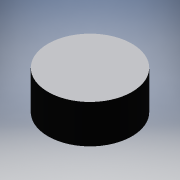
# Autodesk Inventor part: SweepV0.991_BASE_Rev.1
Saved by Autodesk Inventor 2016 (Build 200138000, 138)
## iProperties
Created: 2018-03-01
Part Number: SweepV0.991_BASE_Rev.1
Material: LCP Plastic
Document SubType Name: Modeling
Designer: emvanzant
Density: 1.626 g/cm^3
Appearance: Smooth - White
Author: emvanzant
Autodesk Inventor part; units mm, degrees
ref_plane "YZ Plane" through (0, 0, 0) normal (1, 0, 0) x (0, 1, 0)
sketch "Sketch1" plane through (0, 0, 0) normal (0, 1, 0) x (-1, 0, 0)
  circle A0 centre (0, 0) radius 32.5
  dimension "d0" = 65
  constraints: 1 centre point, 1 coincident
  measures "d0" diameter of A0
extrude "Extrusion1" add sketch "Sketch1" along normal blind 38.5
sketch "Sketch2" plane through (0, 0, 0) normal (0, -1, 0) x (1, 0, 0)
  circle A0 centre (0, 0) radius 25.5
  dimension "d3" = 51
  constraints: 1 centre point, 1 coincident
  measures "d3" diameter of A0
extrude "Extrusion2" add sketch "Sketch2" along normal blind 23.4
chamfer "Chamfer1" distance 3 angle 45 2 edges at (32.5, 38.5, 0) (32.5, 0, 0)
sketch "Sketch3" plane through (0, -23.4, 0) normal (0, -1, 0) x (1, 0, 0)
  line L0 (0, 0) -> (0, -10.5) construction
  circle A0 centre (0, 0) radius 25.5 projected
  line L1 (0, -10.5) -> (5.75, -10.5)
  line L2 (5.75, -10.5) -> (5.75, -24.8433)
  line L3 (0, -10.5) -> (-5.75, -10.5)
  line L4 (-5.75, -10.5) -> (-5.75, -24.8433)
  line L5 (5.75, -24.8433) -> (-5.75, -24.8433)
  line L6 (-15, 15) -> (15, 15) construction
  line L7 (15, 15) -> (15, -15) construction
  line L8 (15, -15) -> (-15, -15) construction
  line L9 (-15, -15) -> (-15, 15) construction
  line L10 (-15, 15) -> (15, -15) construction
  line L11 (15, 15) -> (-15, -15) construction
  line L12 (5.65, 5.65) -> (-5.65, 5.65) construction
  line L13 (-5.65, 5.65) -> (-5.65, -5.65) construction
  line L14 (-5.65, -5.65) -> (5.65, -5.65) construction
  line L15 (5.65, -5.65) -> (5.65, 5.65) construction
  line L16 (5.65, 5.65) -> (-5.65, -5.65) construction
  line L17 (-5.65, 5.65) -> (5.65, -5.65) construction
  dimension "d10" = 10.5
  dimension "d14" = 5.75
  dimension "d15" = 5.75
  dimension "d16" = 30
  dimension "d17" = 30
  dimension "d35" = 11.3
  dimension "d36" = 11.3
  constraints: 36 end point, 8 coincident, 4 horizontal, 4 midpoint, 4 parallel, 4 perpendicular, 2 point on circle, 1 vertical
  measures "d10" distance of L0.start L0.end
  measures "d14" distance of L0.end L1.end
  measures "d15" distance of L0.end L3.end
  measures "d16" distance of L7.end L8.end
  measures "d17" distance of L6.end L7.end
  measures "d35" distance of L14.end L13.end
  measures "d36" distance of L13.end L12.end
hole "Hole1" at (15, -23.4, -15) at (-15, -23.4, -15) at (15, -23.4, 15) at (-15, -23.4, 15) direction (0, 1, 0) diameter 2.5 depth 4
thread "Thread1" size "M2.5x0.45" class "6H" standard "ANSI Metric M Profile" full length
thread "Thread2" size "M2.5x0.45" class "6H" standard "ANSI Metric M Profile" full length
thread "Thread3" size "M2.5x0.45" class "6H" standard "ANSI Metric M Profile" full length
thread "Thread4" size "M2.5x0.45" class "6H" standard "ANSI Metric M Profile" full length
extrude "Extrusion3" cut sketch "Sketch3" against normal blind 12 contours L5 A0 | L4 L3 L1 L2 L5
hole "Hole2" at (5.65, -23.4, 5.65) at (5.65, -23.4, -5.65) at (-5.65, -23.4, 5.65) at (-5.65, -23.4, -5.65) direction (0, 1, 0) diameter 2.1 depth 3 tip angle 118
thread "Thread5" size "M2.5x0.45" class "6H" standard "ANSI Metric M Profile" full length
thread "Thread6" size "M2.2x0.45" class "6H" standard "ANSI Metric M Profile" full length
thread "Thread7" size "M2.2x0.45" class "6H" standard "ANSI Metric M Profile" full length
thread "Thread8" size "M2.2x0.45" class "6H" standard "ANSI Metric M Profile" full length
ref_plane "Work Plane1" through (0, 0, -32.5) normal (0, 0, -1) x (-1, 0, 0)
sketch "Sketch4" plane through (0, 0, -32.5) normal (0, 0, -1) x (-1, 0, 0)
  line L0 (-25.5, -23.4) -> (25.5, -23.4) projected
  line L1 (-32.5, 3) -> (32.5, 3) projected
  line L2 (32.5, 35.5) -> (-32.5, 35.5) projected
  line L3 (0, -23.4) -> (0, 18.1) construction
  line L4 (32.5, 3) -> (32.5, 35.5) projected
  line L5 (-32.5, 3) -> (-32.5, 35.5) projected
  line L6 (-32.5, 17.6) -> (32.5, 17.6)
  line L7 (32.5, 17.6) -> (32.5, 18.6)
  line L8 (32.5, 18.6) -> (-32.5, 18.6)
  line L9 (-32.5, 18.6) -> (-32.5, 17.6)
  line L10 (-32.5, 17.6) -> (32.5, 18.6) construction
  line L11 (32.5, 17.6) -> (-32.5, 18.6) construction
  line L12 (-20, 18.1) -> (20, 18.1) construction
  line L13 (-20, 9.1) -> (20, 9.1)
  line L14 (20, 27.1) -> (-20, 27.1)
  arc A0 (-20, 27.1) -> (-20, 9.1) centre (-20, 18.1) ccw
  arc A1 (20, 9.1) -> (20, 27.1) centre (20, 18.1) ccw
  line L15 (0, 18.1) -> (-15, 18.1)
  line L16 (0, 18.1) -> (15, 18.1)
  circle A2 centre (-15, 18.1) radius 6.35
  circle A3 centre (15, 18.1) radius 6.35
  line L17 (-20, 25.6) -> (20, 25.6)
  arc A4 (20, 10.6) -> (20, 25.6) centre (20, 18.1) ccw
  line L18 (20, 10.6) -> (-20, 10.6)
  arc A5 (-20, 25.6) -> (-20, 10.6) centre (-20, 18.1) ccw
  point P0 (0, 0)
  point P1 (-5.75, -23.4)
  point P2 (5.75, -23.4)
  dimension "d52" = 41.5
  dimension "d53" = 1
  dimension "d54" = 20
  dimension "d55" = 18
  dimension "d56" = 15
  dimension "d57" = 15
  dimension "d58" = 12.7
  dimension "d59" = 12.7
  dimension "d64" = 1.5
  constraints: 30 end point, 8 point on circle, 6 centre point, 5 parallel, 4 midpoint, 4 tangent, 2 coincident, 2 perpendicular, 2 point on line, 1 vertical, 3 other
  measures "d52" distance of L3.start L3.end
  measures "d53" distance of L7.end L6.end
  measures "d54" distance of L3.end L12.end
  measures "d55" diameter of A1
  measures "d56" distance of L3.end L15.end
  measures "d57" distance of L3.end L16.end
  measures "d58" diameter of A2
  measures "d59" diameter of A3
  measures "d64" distance between parallel lines of L14 L17
extrude "Extrusion5" cut sketch "Sketch4" against normal blind 15 contours A2 L8 L6 | L6 A2 | A3 L6 | L6 A3 L8 | A2 L8 | L8 A3
sketch "Sketch5" plane through (0, 0, 0) normal (1, 0, 0) x (0, 1, 0)
  line L0 (3, -32.5) -> (35.5, -32.5) projected
  line L1 (18.6, -33) -> (17.6, -33)
  line L2 (17.6, -33) -> (17.6, -32)
  line L3 (17.6, -32) -> (18.6, -32)
  line L4 (18.6, -32) -> (18.6, -33)
  line L5 (18.6, -33) -> (17.6, -32) construction
  line L6 (17.6, -33) -> (18.6, -32) construction
  line L7 (-35.78, 0) -> (50.88, 0) projected
  point P0 (0, 0)
  point P1 (18.1, -32.5)
  point P2 (18.1, -32.5)
  point P3 (18.1, -32.5)
  dimension "d67" = 1
  dimension "d68" = 1
  constraints: 12 end point, 2 midpoint, 2 parallel, 1 horizontal, 1 perpendicular
  measures "d67" distance of L2.end L3.end
  measures "d68" distance of L1.end L2.end
revolve "Revolution1" cut sketch "Sketch5" angle 360 about axis through (0, -10, 0) along (0, 1, 0)
ref_plane "Work Plane2" through (0, 0, 0) normal (0, -1, 0) x (1, 0, 0)
split "Split1" plane through (0, 0, 0) removes the side toward (0, 1, 0)
sketch "Sketch6" plane through (0, 0, 0) normal (0, 1, 0) x (1, 0, 0)
  point P0 (0, 0)
body "Solid1"
